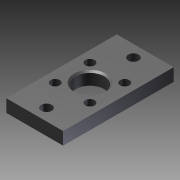
# Autodesk Inventor part: 537247 FNC-20---(F)
Saved by Autodesk Inventor 2011 SP1 (Build 150282100, 282)
## iProperties
Created: 2018-05-29
Part Number: 537247 FNC-20---(F)
Catalog Web Link: www.cadenas.de
Description: FNC-(F)-Flange mounting
Vendor: FESTO
Document SubType Name: Modeling
Designer: psAdmin
Manufacturer: FESTO
Mass: 15.6597 g
Surface Area: 74.7814 cm^2
Volume: 15.6597 cm^3
Density: 1 g/cm^3
Category: PARTsolutions
Company: FESTO
Title: 537247 FNC-20
Author: Cadenas PARTsolutions
Comments: Flange mounting
PSOL_IDENT_0: {$CADENAS_DATA\23d-libs\festo\parts\f\fnc\fnc.prj},176 {VTYP=3D},{NB=537247 FNC-20---(F)},{LINA=5372
PSOL_IDENT_1: 47 FNC-20},{NN=FNC-(F)},{DATE=13.11.2017 12:35:20},{GEOMDATE=13.11.2017 12:34:23},{VERSION=},{LINEID=
PSOL_IDENT_2: 110},{LINESUBID=-1},{WBVAR=}  {NB=537247 FNC-20---(F)},{LINA=537247 FNC-20},{KT=DUMMY},{TNR=537247},
PSOL_IDENT_3: {TYP=FNC-20},{VERS=1},{D1=18.000},{D2=5.800},{D3=10.000},{E=36.000},{F=1.000},{FB=6.600},{MF=8.000},
PSOL_IDENT_4: {R=0.000},{T=3.000},{TF=55.000},{TG1=22.000},{UF=70.000},{ZZ=0},{DK=20},{D6912D=5.000},{D6912L=20.00
PSOL_IDENT_5: 0}
NN: FNC-(F)
NT: Flange mounting
NB: 537247 FNC-20---(F)
NBSYN: $TNR. $TYP.---(F)
LINA: 537247 FNC-20
TNR: 537247
TYP: FNC-20
D1: 18.000
D2: 5.800
D3: 10.000
E: 36.000
F: 1.000
FB: 6.600
MF: 8.000
R: 0.000
T: 3.000
TF: 55.000
TG1: 22.000
UF: 70.000
SUPPLIER: FESTO
ARTICLENO: 537247 FNC-20---(F)
BOMINFO: 537247 FNC-20
CREATOR: CADENAS GmbH
Autodesk Inventor part; units mm, degrees
sketch "Skizze_1" plane through (0, 0, 0) normal (0, 0, 1) x (1, 0, 0)
  line L0 (-18, 35) -> (-18, -35)
  line L1 (-18, -35) -> (18, -35)
  line L2 (18, -35) -> (18, 35)
  line L3 (18, 35) -> (-18, 35)
  circle A0 centre (0, 27.5) radius 3.3
  circle A1 centre (0, -27.5) radius 3.3
  constraints: 8 end point, 2 centre point
extrude "Extrusion1" add sketch "Skizze_1" along normal blind 8
sketch "Skizze_2_ALT_Drilling_1" plane through (0, 0, 0) normal (1, 0, 0) x (0, 1, 0)
  line L0 (0, 0) -> (0, 8)
  line L1 (0, 8) -> (10, 8)
  line L2 (10, 8) -> (9, 7)
  line L3 (9, 7) -> (9, 0)
  line L4 (9, 0) -> (0, 0)
  line L5 (0, 0) -> (0, 8)
  constraints: 12 end point
revolve "Revolution1" cut sketch "Skizze_2_ALT_Drilling_1" angle 360 about axis through (0, 0, 0) along (0, 0, -1)
sketch "Skizze_3_ALT_Drilling_2" plane through (11, 0, 0) normal (1, 0, 0) x (0, 0, -1)
  line L0 (0, 11) -> (-8, 11)
  line L1 (-8, 11) -> (-8, 13.9)
  line L2 (-8, 13.9) -> (-5, 13.9)
  line L3 (-5, 13.9) -> (-5, 16)
  line L4 (-5, 16) -> (0, 16)
  line L5 (0, 16) -> (0, 11)
  line L6 (0, 11) -> (-8, 11)
  constraints: 14 end point
revolve "Revolution2" cut sketch "Skizze_3_ALT_Drilling_2" angle 360 about axis through (11, 11, 0) along (0, 0, -1)
sketch "Muster_1_SKETCH_1" plane through (-11, 0, 0) normal (1, 0, 0) x (0, 0, -1)
  line L0 (0, 11) -> (-8, 11)
  line L1 (-8, 11) -> (-8, 13.9)
  line L2 (-8, 13.9) -> (-5, 13.9)
  line L3 (-5, 13.9) -> (-5, 16)
  line L4 (-5, 16) -> (0, 16)
  line L5 (0, 16) -> (0, 11)
  line L6 (0, 11) -> (-8, 11)
  constraints: 14 end point
sketch "Muster_1_SKETCH_2" plane through (11, 0, 0) normal (1, 0, 0) x (0, 0, -1)
  line L0 (0, -11) -> (-8, -11)
  line L1 (-8, -11) -> (-8, -8.1)
  line L2 (-8, -8.1) -> (-5, -8.1)
  line L3 (-5, -8.1) -> (-5, -6)
  line L4 (-5, -6) -> (0, -6)
  line L5 (0, -6) -> (0, -11)
  line L6 (0, -11) -> (-8, -11)
  constraints: 14 end point
sketch "Muster_1_SKETCH_3" plane through (-11, 0, 0) normal (1, 0, 0) x (0, 0, -1)
  line L0 (0, -11) -> (-8, -11)
  line L1 (-8, -11) -> (-8, -8.1)
  line L2 (-8, -8.1) -> (-5, -8.1)
  line L3 (-5, -8.1) -> (-5, -6)
  line L4 (-5, -6) -> (0, -6)
  line L5 (0, -6) -> (0, -11)
  line L6 (0, -11) -> (-8, -11)
  constraints: 14 end point
revolve "Revolution3" cut sketch "Muster_1_SKETCH_1" angle 360 about axis through (-11, 11, 0) along (0, 0, -1)
revolve "Revolution4" cut sketch "Muster_1_SKETCH_2" angle 360 about axis through (11, -11, 0) along (0, 0, -1)
revolve "Revolution5" cut sketch "Muster_1_SKETCH_3" angle 360 about axis through (-11, -11, 0) along (0, 0, -1)
ref_plane "FDT_MOUNT_XY" through (0, 0, 8) normal (0, 0, 1) x (0, 1, 0)
ref_plane "FDT_MOUNT_YZ" through (0, 0, 8) normal (0, 1, 0) x (-1, 0, 0)
ref_plane "FDT_MOUNT_ZX" through (0, 0, 8) normal (-1, 0, 0) x (0, 0, 1)
ref_plane "FNC_1_XY" through (0, 0, 4) normal (0, 0, 1) x (1, 0, 0)
ref_plane "FNC_1_YZ" through (0, 0, 4) normal (1, 0, 0) x (0, 1, 0)
ref_plane "FNC_1_ZX" through (0, 0, 4) normal (0, 1, 0) x (0, 0, 1)
ref_plane "FNC_2_3_XY" through (0, 0, 8) normal (0, 0, 1) x (1, 0, 0)
ref_plane "FNC_2_3_YZ" through (0, 0, 8) normal (1, 0, 0) x (0, 1, 0)
ref_plane "FNC_2_3_ZX" through (0, 0, 8) normal (0, 1, 0) x (0, 0, 1)
ref_plane "FNC_Schraube_1_XY" through (-11, 11, 5) normal (0, 0, 1) x (1, 0, 0)
ref_plane "FNC_Schraube_1_YZ" through (-11, 11, 5) normal (1, 0, 0) x (0, 1, 0)
ref_plane "FNC_Schraube_1_ZX" through (-11, 11, 5) normal (0, 1, 0) x (0, 0, 1)
ref_plane "FNC_Schraube_2_XY" through (11, 11, 5) normal (0, 0, 1) x (1, 0, 0)
ref_plane "FNC_Schraube_2_YZ" through (11, 11, 5) normal (1, 0, 0) x (0, 1, 0)
ref_plane "FNC_Schraube_2_ZX" through (11, 11, 5) normal (0, 1, 0) x (0, 0, 1)
ref_plane "FNC_Schraube_3_XY" through (-11, -11, 5) normal (0, 0, 1) x (1, 0, 0)
ref_plane "FNC_Schraube_3_YZ" through (-11, -11, 5) normal (1, 0, 0) x (0, 1, 0)
ref_plane "FNC_Schraube_3_ZX" through (-11, -11, 5) normal (0, 1, 0) x (0, 0, 1)
ref_plane "FNC_Schraube_4_XY" through (11, -11, 5) normal (0, 0, 1) x (1, 0, 0)
ref_plane "FNC_Schraube_4_YZ" through (11, -11, 5) normal (1, 0, 0) x (0, 1, 0)
ref_plane "FNC_Schraube_4_ZX" through (11, -11, 5) normal (0, 1, 0) x (0, 0, 1)
ref_plane "P17_1_XY" through (0, 27.5, 8) normal (0, 0, 1) x (1, 0, 0)
ref_plane "P17_1_YZ" through (0, 27.5, 8) normal (1, 0, 0) x (0, 1, 0)
ref_plane "P17_1_ZX" through (0, 27.5, 8) normal (0, 1, 0) x (0, 0, 1)
ref_plane "P18_1_XY" through (0, -27.5, 8) normal (0, 0, 1) x (1, 0, 0)
ref_plane "P18_1_YZ" through (0, -27.5, 8) normal (1, 0, 0) x (0, 1, 0)
ref_plane "P18_1_ZX" through (0, -27.5, 8) normal (0, 1, 0) x (0, 0, 1)
body "Solid1"
